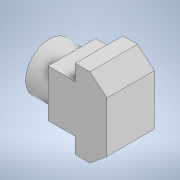
# Autodesk Inventor part: m_Schienenteil
Saved by Autodesk Inventor 2020.3 (Build 243373000, 373)
## iProperties
Created: 2020-10-08
Part Number: m_Schienenteil
Material: Generic
Document SubType Name: Modeling
Designer: Mara
Density: 1 g/cm^3
Appearance: Default
Author: Mara
Autodesk Inventor part; units mm, degrees
ref_plane "YZ Plane" through (0, 0, 0) normal (1, 0, 0) x (0, 1, 0)
ref_plane "XZ Plane" through (0, 0, 0) normal (0, 1, 0) x (-1, 0, 0)
ref_plane "XY Plane" through (0, 0, 0) normal (0, 0, 1) x (1, 0, 0)
sketch "Sketch1" plane through (0, 0, 0) normal (0, 0, 1) x (1, 0, 0)
  line L0 (0, 10.5) -> (12, 10.5)
  line L1 (12, 10.5) -> (12, 17.5)
  line L2 (12, 17.5) -> (18.5, 17.5)
  line L3 (18.5, 17.5) -> (26, 11.2068)
  line L4 (0, 10.5) -> (0, -10.5)
  line L5 (0, -10.5) -> (12, -10.5)
  line L6 (12, -10.5) -> (12, -17.5)
  line L7 (12, -17.5) -> (18.5, -17.5)
  line L8 (18.5, -17.5) -> (26, -11.2068)
  line L9 (26, -11.2068) -> (26, 11.2068)
  point P0 (0, 0)
  point P1 (0, 0)
  dimension "d0" = 12
  dimension "d1" = 7
  dimension "d2" = 6.5
  dimension "d3" = 21
  dimension "d5" = 14
  dimension "d8" = 140
  dimension "d9" = 140
  constraints: 20 end point, 4 perpendicular, 3 equal length, 2 horizontal, 2 vertical, 1 coincident, 1 midpoint
  measures "d0" distance of L0.start L0.end
  measures "d1" distance of L0.end L1.end
  measures "d2" distance of L1.end L2.end
  measures "d3" distance of L0.start L4.end
  measures "d5" horizontal distance of L3.end L0.end
  measures "d8" angle of L2 L3
  measures "d9" angle of L7 L8
extrude "Extrusion1" add sketch "Sketch1" along normal blind 21
sketch "Sketch2" plane through (0, -10.5, 0) normal (-1, 0, 0) x (0, 0, 1)
  line L0 (0, 21) -> (0, 0) projected
  line L1 (0, 21) -> (0, 0) projected
  line L2 (0, 0) -> (21, 0) projected
  line L3 (21, 21) -> (21, 0) projected
  line L4 (0, 21) -> (21, 21) projected
  circle A0 centre (10.5, 10.5) radius 10.5
  point P0 (0, 10.5)
  constraints: 3 tangent, 1 centre point
extrude "Extrusion2" add sketch "Sketch2" along normal blind 10 contours A0
equation "\"d9\" = d8"
body "Solid1"
